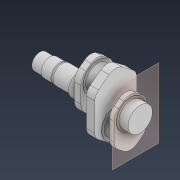
# Autodesk Inventor part: Korbowód poprawiony
Saved by Autodesk Inventor 2022 (Build 260153000, 153)
## iProperties
Created: 2023-04-16
Part Number: Korbowód poprawiony
Material: Generic
Document SubType Name: Modeling
Designer: wikto
Density: 1 g/cm^3
Appearance: Default
Author: wikto
Autodesk Inventor part; units mm, degrees
ref_plane "YZ Plane" through (0, 0, 0) normal (1, 0, 0) x (0, 1, 0)
sketch "Sketch1" plane through (0, 0, 0) normal (0, 0, 1) x (1, 0, 0)
  line L0 (0, 0) -> (115.5, 0)
  line L1 (0, 0) -> (0, 18)
  line L2 (0, 18) -> (23, 18)
  line L3 (23, 18) -> (23, 20)
  line L4 (23, 20) -> (46, 20)
  line L5 (46, 20) -> (46, 21)
  line L6 (46, 21) -> (48, 21)
  arc A0 (48, 21) -> (51, 21) centre (49.5, 21) ccw
  line L7 (51, 21) -> (90, 21)
  line L8 (90, 21) -> (90, 25)
  line L9 (115.5, 32.5) -> (115.5, 0)
  line L10 (90, 25) -> (114.5, 25)
  line L11 (114.5, 25) -> (114.5, 32.5)
  line L12 (114.5, 32.5) -> (115.5, 32.5)
  dimension "d1" = 23
  dimension "d2" = 23
  dimension "d3" = 44
  dimension "d4" = 36
  dimension "d6" = 40
  dimension "d7" = 42
  dimension "d9" = 25.5
  dimension "d10" = 2
  dimension "d11" = 1.5
  dimension "d13" = 65
  dimension "d14" = 50
  dimension "d15" = 1
  constraints: 26 end point, 8 perpendicular, 3 horizontal, 3 horizontal alignment, 2 point on circle, 1 centre point, 1 vertical
  measures "d1" distance between parallel lines of L3 L1
  measures "d2" distance between parallel lines of L5 L3
  measures "d3" distance between parallel lines of L8 L5
  measures "d4" diameter of L2 L0
  measures "d6" diameter of L4 L0
  measures "d7" diameter of L7 L0
  measures "d9" distance between parallel lines of L8 L9
  measures "d10" distance of L5.end L6.end
  measures "d11" radius of A0
  measures "d13" diameter of L12 L0
  measures "d14" diameter of L10 L0
  measures "d15" distance between parallel lines of L9 L11
revolve "Revolution1" add sketch "Sketch1" angle 360 about axis through (0, 0, 0) along (1, 0, 0)
ref_plane "Work Plane7" through (130.26, 0, 0) normal (1, 0, 0) x (0, 0, -1)
sketch "Sketch22" plane through (130.26, 0, 0) normal (1, 0, 0) x (0, 0, -1)
  circle A0 centre (0, 34.5) radius 32.5
  circle A1 centre (0, 34.5) radius 27.5
  point P0 (0, 0)
  dimension "d97" = 65
  dimension "d98" = 55
  dimension "d99" = 34.5
  constraints: 2 centre point, 1 coincident, 1 vertical alignment
  measures "d97" diameter of A0
  measures "d98" diameter of A1
  measures "d99" distance of point (0, 0) A0.centre
extrude "Extrusion18" add sketch "Sketch22" along normal blind 22 contours A1
extrude "Extrusion19" add sketch "Sketch22" along normal blind 1
sketch "Sketch23" plane through (115.5, 0, 0) normal (1, 0, 0) x (0, 0, -1)
  line L0 (-37, -1.125) -> (-37, 35.625)
  line L1 (37, -1.125) -> (37, 35.625)
  arc A0 (-37, -1.125) -> (-25.6, -23.925) centre (-8.5, -1.125) ccw
  arc A1 (25.6, -23.925) -> (37, -1.125) centre (8.5, -1.125) ccw
  line L2 (-25.6, -23.925) -> (-13.6, -32.925)
  line L3 (25.6, -23.925) -> (13.6, -32.925)
  arc A2 (-13.6, -32.925) -> (13.6, -32.925) centre (0, -14.7917) ccw
  line L4 (4.9524, -36.9107) -> (32.7905, -16.0321) construction
  circle A3 centre (0, 0) radius 32.5 projected
  line L5 (-37, 17.25) -> (37, 17.25) construction
  arc A4 (-25.6, 58.425) -> (-37, 35.625) centre (-8.5, 35.625) ccw
  arc A5 (37, 35.625) -> (25.6, 58.425) centre (8.5, 35.625) ccw
  line L6 (-25.6, 58.425) -> (-13.6, 67.425)
  line L7 (25.6, 58.425) -> (13.6, 67.425)
  arc A6 (13.6, 67.425) -> (-13.6, 67.425) centre (0, 49.2917) ccw
  line L8 (4.9524, 71.4107) -> (32.7905, 50.5321) construction
  circle A7 centre (0, 34.5) radius 32.5 construction
  dimension "d105" = 15
  dimension "d106" = 74
  dimension "d107" = 27.2
  dimension "d108" = 51.2
  dimension "d109" = 2
  dimension "d126" = 2
  constraints: 18 end point, 16 point on circle, 8 tangent, 7 symmetric about line, 6 centre point, 4 horizontal alignment, 2 midpoint, 2 parallel, 2 vertical, 1 vertical alignment, 3 other
  measures "d105" distance of L2.start L2.end
  measures "d106" distance between parallel lines of L1 L0
  measures "d107" distance of L3.end L2.end
  measures "d108" distance of L3.start L2.start
  measures "d109" distance between parallel lines of L4 L3
  measures "d126" distance between parallel lines of L7 L8
extrude "Extrusion20" add sketch "Sketch23" along normal up to surface (14.76 mm away) contours L0 A4 L6 A6 L7 A5 L1 A1 L3 A2 L2 A0 | A3
sketch "Sketch24" plane through (152.26, 34.5, 0) normal (1, 0, 0) x (0, 0, -1)
  circle A0 centre (0, 0) radius 32.5 projected
  point P0 (0, -34.5)
extrude "Extrusion21" add sketch "Sketch24" along normal blind 1
ref_plane "Work Plane8" through (172.17, 34.5, 0) normal (1, 0, 0) x (0, 0, -1)
sketch "Sketch25" plane through (172.17, 34.5, 0) normal (1, 0, 0) x (0, 0, -1)
  circle A0 centre (0, -69) radius 32.5
  circle A1 centre (0, 0) radius 32.5 construction
  point P0 (0, -34.5)
  dimension "d115" = 65
  dimension "d116" = 69
  constraints: 1 centre point, 1 vertical alignment
  measures "d115" diameter of A0
  measures "d116" distance of A0.centre A1.centre
extrude "Extrusion22" add sketch "Sketch25" along normal blind 1
sketch "Sketch26" plane through (153.26, 34.5, 0) normal (1, 0, 0) x (0, 0, -1)
  arc A0 (15, 32.4583) -> (-15, 32.4583) centre (0, 12.4583) ccw
  line L0 (-15, 32.4583) -> (-38.92, 14.5183)
  line L1 (15, 32.4583) -> (38.92, 14.5183)
  arc A1 (47.5, -2.6417) -> (38.92, 14.5183) centre (26.05, -2.6417) ccw
  arc A2 (-38.92, 14.5183) -> (-47.5, -2.6417) centre (-26.05, -2.6417) ccw
  line L2 (-47.5, -2.6417) -> (-47.5, -65.775)
  line L3 (47.5, -2.6417) -> (47.5, -65.775)
  arc A3 (13.6, 32.925) -> (-13.6, 32.925) centre (0, 14.7917) ccw projected
  line L4 (-47.5, -34.2083) -> (47.5, -34.2083) construction
  line L5 (13.6, 32.925) -> (25.6, 23.925) projected
  arc A4 (-15, -100.875) -> (15, -100.875) centre (0, -80.875) ccw
  line L6 (-15, -100.875) -> (-38.92, -82.935)
  line L7 (15, -100.875) -> (38.92, -82.935)
  arc A5 (38.92, -82.935) -> (47.5, -65.775) centre (26.05, -65.775) ccw
  arc A6 (-47.5, -65.775) -> (-38.92, -82.935) centre (-26.05, -65.775) ccw
  line L8 (5.9616, -105.1538) -> (30.4845, -86.7616) construction
  circle A7 centre (0, -69) radius 32.5 projected
  point P0 (0, -34.5)
  point P1 (0, 37.4583)
  dimension "d119" = 25
  dimension "d120" = 29.9
  dimension "d122" = 95
  dimension "d127" = 2
  constraints: 16 end point, 16 point on circle, 7 symmetric about line, 7 tangent, 6 centre point, 4 horizontal alignment, 2 midpoint, 2 parallel, 2 vertical, 1 vertical alignment, 3 other
  measures "d119" radius of A0
  measures "d120" distance of L1.start L1.end
  measures "d122" distance between parallel lines of L3 L2
  measures "d127" distance between parallel lines of L8 L7
extrude "Extrusion23" add sketch "Sketch26" along normal up to surface (18.91 mm away) contours L1 A1 L3 A5 L7 A4 L6 A6 L2 A2 L0 A0 | A7
sketch "Sketch27" plane through (173.17, -34.5, 0) normal (1, 0, 0) x (0, 0, -1)
  circle A0 centre (0, 0) radius 27.5
  circle A1 centre (0, 0) radius 32.5 projected
  point P0 (0, 34.5)
  dimension "d128" = 55
  constraints: 1 centre point, 1 coincident
  measures "d128" diameter of A0
extrude "Extrusion24" add sketch "Sketch27" along normal blind 21 contours A0
sketch "Sketch28" plane through (194.17, -34.5, 0) normal (1, 0, 0) x (0, 0, -1)
  circle A0 centre (0, 0) radius 32.5 projected
  point P0 (0, 34.5)
extrude "Extrusion25" add sketch "Sketch28" along normal blind 1
sketch "Sketch29" plane through (195.17, -34.5, 0) normal (1, 0, 0) x (0, 0, -1)
  arc A0 (-15, -31.875) -> (15, -31.875) centre (0, -11.875) ccw projected
  line L0 (-15, -31.875) -> (-27, -22.875)
  line L1 (38.92, -13.935) -> (15, -31.875) construction
  line L2 (15, -31.875) -> (27, -22.875)
  line L3 (-15, -31.875) -> (-38.92, -13.935) construction
  arc A1 (27, -22.875) -> (37, -2.875) centre (12, -2.875) ccw
  arc A2 (-37, -2.875) -> (-27, -22.875) centre (-12, -2.875) ccw
  line L4 (-37, -2.875) -> (-37, 37.525)
  line L5 (37, -2.875) -> (37, 37.525)
  arc A3 (-27, 57.525) -> (-37, 37.525) centre (-12, 37.525) ccw
  arc A4 (37, 37.525) -> (27, 57.525) centre (12, 37.525) ccw
  line L6 (-27, 57.525) -> (-15, 66.525)
  line L7 (27, 57.525) -> (15, 66.525)
  arc A5 (15, 66.525) -> (-15, 66.525) centre (0, 46.525) ccw
  point P0 (0, 34.5)
  dimension "d133" = 15
  dimension "d134" = 25
  dimension "d135" = 40.4
  dimension "d136" = 25
  constraints: 13 end point, 10 point on circle, 8 tangent, 5 centre point, 4 horizontal alignment, 3 equal radius, 2 collinear, 2 equal length, 2 vertical
  measures "d133" distance of L0.start L0.end
  measures "d134" radius of A1
  measures "d135" distance of L5.start L5.end
  measures "d136" radius of A4
extrude "Extrusion26" add sketch "Sketch29" along normal blind 10.43
sketch "Sketch30" plane through (205.6, -34.5, 0) normal (1, 0, 0) x (0, 0, -1)
  circle A0 centre (0, 34.5) radius 18 construction
  circle A1 centre (0, 34.5) radius 32.5
  dimension "d139" = 65
  constraints: 1 centre point, 1 coincident
  measures "d139" diameter of A1
extrude "Extrusion27" add sketch "Sketch30" along normal blind 1
sketch "Sketch31" plane through (206.6, 0, 0) normal (1, 0, 0) x (0, 0, -1)
  circle A0 centre (0, 0) radius 27.5
  dimension "d142" = 55
  constraints: 1 centre point, 1 coincident
  measures "d142" diameter of A0
extrude "Extrusion28" add sketch "Sketch31" along normal blind 21
ref_plane "Work Plane9" through (217.1, 0, 0) normal (1, 0, 0) x (0, 0, -1)
body "Solid1"
